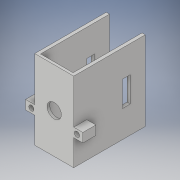
# Autodesk Inventor part: motor_mount
Saved by Autodesk Inventor 2019.5 (Build 235369000, 369)
## iProperties
Created: 2021-07-19
Part Number: motor_mount
Material: Generisch
Document SubType Name: Modeling
Designer: c-man
Density: 1 g/cm^3
Appearance: Vorgabe
Author: c-man
Autodesk Inventor part; units mm, degrees
ref_plane "YZ Plane" through (0, 0, 0) normal (1, 0, 0) x (0, 1, 0)
ref_plane "XZ Plane" through (0, 0, 0) normal (0, 1, 0) x (-1, 0, 0)
ref_plane "XY Plane" through (0, 0, 0) normal (0, 0, 1) x (1, 0, 0)
sketch "Skizze1" plane through (0, 0, 0) normal (0, 0, 1) x (1, 0, 0)
  line L0 (0, 0) -> (0, 61)
  line L1 (25, 0) -> (25, 61)
  line L2 (0, 61) -> (-2.5, 61)
  line L3 (25, 61) -> (27.5, 61)
  line L4 (-2.5, 61) -> (-2.5, 0)
  line L5 (-2.5, 0) -> (0, 0)
  line L6 (27.5, 61) -> (27.5, 0)
  line L7 (27.5, 0) -> (25, 0)
  dimension "d1" = 61
  dimension "d2" = 61
  dimension "d3" = 25
  dimension "d4" = 2.5
  dimension "d5" = 2.5
  constraints: 16 end point, 4 vertical, 2 horizontal, 2 perpendicular
  measures "d1" distance of L1.start L1.end
  measures "d2" distance of L0.start L0.end
  measures "d3" distance between parallel lines of L1 L0
  measures "d4" distance of L0.end L2.end
  measures "d5" distance of L1.end L3.end
extrude "Extrusion1" add sketch "Skizze1" along normal blind 55
sketch "Skizze2" plane through (0, 0, 0) normal (1, 0, 0) x (0, 0, -1)
  line L0 (-55, 61) -> (-55, 0) projected
  line L1 (0, 0) -> (-55, 0) projected
  line L2 (-55, 61) -> (-53, 61)
  line L3 (-53, 61) -> (-53, 0)
  line L4 (-53, 0) -> (-55, 0)
  line L5 (-55, 0) -> (-55, 61)
  dimension "d8" = 2
  constraints: 8 end point, 2 parallel, 1 horizontal, 1 perpendicular, 1 point on line
  measures "d8" distance of L0.start L2.end
extrude "Extrusion2" add sketch "Skizze2" along normal blind 25
sketch "Skizze3" plane through (0, 0, 55) normal (0, 0, 1) x (1, 0, 0)
  circle A0 centre (12.5, 30.5) radius 5.5
  line L0 (27.5, 61) -> (-2.5, 61) projected
  line L1 (27.5, 0) -> (27.5, 61) projected
  line L2 (27.5, 61) -> (27.5, 0) projected
  line L3 (27.5, 0) -> (-2.5, 0) projected
  line L4 (-2.5, 0) -> (-2.5, 61) projected
  line L5 (-2.5, 61) -> (27.5, 61) projected
  line L6 (27.5, 61) -> (-2.5, 61) projected
  line L7 (-2.5, 61) -> (-2.5, 0) projected
  line L8 (-2.5, 0) -> (27.5, 0) projected
  line L9 (27.5, 0) -> (27.5, 61) projected
  point P0 (0, 0)
  dimension "d11" = 30.5
  dimension "d12" = 15
  dimension "d13" = 11
  constraints: 1 centre point
  measures "d11" distance from line of L0 A0.centre
  measures "d12" distance from line of L1 A0.centre
  measures "d13" diameter of A0
extrude "Extrusion3" cut sketch "Skizze3" against normal blind 2.5 contours A0
sketch "Skizze4" plane through (0, 0, 55) normal (0, 0, 1) x (1, 0, 0)
  circle A0 centre (12.5, 30.5) radius 5.5 projected
  line L0 (27.5, 61) -> (27.5, 0) projected
  line L1 (27.5, 0) -> (-2.5, 0) projected
  line L2 (-2.5, 0) -> (-2.5, 61) projected
  line L3 (-2.5, 61) -> (27.5, 61) projected
  circle A1 centre (12.5, 30.5) radius 5.5 projected
  line L4 (27.5, 61) -> (27.5, 0) projected
  line L5 (27.5, 0) -> (-2.5, 0) projected
  line L6 (-2.5, 0) -> (-2.5, 61) projected
  line L7 (-2.5, 61) -> (27.5, 61) projected
  circle A2 centre (12.5, 30.5) radius 5.5 projected
  line L8 (27.5, 61) -> (27.5, 0) projected
  line L9 (27.5, 0) -> (-2.5, 0) projected
  line L10 (-2.5, 0) -> (-2.5, 61) projected
  line L11 (-2.5, 61) -> (27.5, 61) projected
  line L12 (-9.5, 27) -> (-9.5, 20)
  line L13 (34.5, 27) -> (34.5, 20)
  line L14 (27.5, 61) -> (27.5, 0) projected
  line L15 (-2.5, 61) -> (-2.5, 0) projected
  line L16 (-9.5, 27) -> (-2.5, 27)
  line L17 (27.5, 27) -> (34.5, 27)
  line L18 (-9.5, 20) -> (-2.5, 20)
  line L19 (27.5, 20) -> (34.5, 20)
  line L20 (-2.5, 20) -> (-2.5, 27)
  line L21 (27.5, 27) -> (27.5, 20)
  point P0 (0, 0)
  dimension "d29" = 7
  dimension "d30" = 7
  dimension "d31" = 7
  dimension "d32" = 7
  constraints: 16 end point, 4 horizontal, 4 point on line, 2 collinear
  measures "d29" distance of L17.start L13.start
  measures "d30" distance of L19.start L13.end
  measures "d31" distance of L12.start L16.end
  measures "d32" distance of L12.end L18.end
extrude "Extrusion4" add sketch "Skizze4" against normal blind 10 contours L17 L13 L19 L0 | L2 L18 L12 L16
sketch "Skizze5" plane through (0, 0, 55) normal (0, 0, 1) x (1, 0, 0)
  circle A0 centre (-5, 23.5) radius 1.9403
  circle A1 centre (30, 23.5) radius 2.0247
  circle A2 centre (12.5, 30.5) radius 5.5 projected
  dimension "d25" = 35
  dimension "d27" = 7
  dimension "d28" = 7
  dimension "d33" = 17.5
  constraints: 2 centre point
  measures "d25" distance of A1.centre A0.centre
  measures "d27" vertical distance of A0.centre A2.centre
  measures "d28" vertical distance of A2.centre A1.centre
  measures "d33" horizontal distance of A1.centre A2.centre
extrude "Extrusion5" cut sketch "Skizze5" against normal blind 10 contours A0 | A1
sketch "Skizze6" plane through (27.5, 0, 0) normal (1, 0, 0) x (0, 0, -1)
  line L0 (-17.5, 40.25) -> (-11.5, 40.25)
  line L1 (-11.5, 40.25) -> (-11.5, 20.75)
  line L2 (-11.5, 20.75) -> (-17.5, 20.75)
  line L3 (-17.5, 20.75) -> (-17.5, 40.25)
  line L4 (0, 61) -> (0, 0) projected
  line L5 (0, 0) -> (-55, 0) projected
  line L6 (-55, 27) -> (-45, 27) projected
  line L7 (-45, 27) -> (-45, 20) projected
  line L8 (-45, 20) -> (-55, 20) projected
  line L9 (-55, 0) -> (-55, 20) projected
  line L10 (0, 0) -> (-55, 0) projected
  line L11 (0, 61) -> (0, 0) projected
  line L12 (0, 61) -> (-55, 61) projected
  line L13 (-55, 27) -> (-55, 61) projected
  point P0 (-17.5, 30.5)
  dimension "d36" = 6
  dimension "d37" = 19.5
  dimension "d38" = 11.5
  dimension "d40" = 30.5
  constraints: 8 end point, 2 parallel, 1 horizontal, 1 midpoint, 1 perpendicular
  measures "d36" distance of L0.start L0.end
  measures "d37" distance of L0.end L1.end
  measures "d38" distance between parallel lines of L4 L1
  measures "d40" distance from line of L5 point (-17.5, 30.5)
extrude "Extrusion6" cut sketch "Skizze6" against normal blind 30 contours L0 L1 L2 L3
sketch "Skizze8" plane through (0, 0, 0) normal (0, 0, -1) x (-1, 0, 0)
  line L0 (0, 20.75) -> (0, 40.25) projected
  line L1 (1, 35.5) -> (0, 35.5)
  line L2 (0, 35.5) -> (0, 25.5)
  line L3 (0, 25.5) -> (1, 25.5)
  line L4 (1, 25.5) -> (1, 35.5)
  line L5 (0, 61) -> (2.5, 61) projected
  line L6 (-25, 0) -> (-25, 61) projected
  line L7 (-25, 35.5) -> (-26, 35.5)
  line L8 (-26, 35.5) -> (-26, 25.5)
  line L9 (-26, 25.5) -> (-25, 25.5)
  line L10 (-25, 25.5) -> (-25, 35.5)
  point P0 (0, 0)
  point P1 (1, 30.5)
  point P2 (13.2784, 51.1394)
  dimension "d43" = 1
  dimension "d44" = 10
  dimension "d45" = 30.5
  dimension "d46" = 1
  constraints: 16 end point, 4 parallel, 2 horizontal, 2 perpendicular, 2 point on line, 1 midpoint
  measures "d43" distance of L2.end L3.end
  measures "d44" distance of L1.end L2.end
  measures "d45" distance from line of L5 point (1, 30.5)
  measures "d46" distance of L8.end L9.end
extrude "Extrusion7" cut sketch "Skizze8" against normal blind 5
